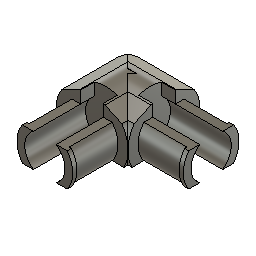
2x corner new v16 (Autodesk Fusion 360 design; units mm, degrees)
Autodesk Fusion 360 part; units mm, degrees
sketch "Sketch7" plane through (0, 0, 0) normal (0, 1, 0) x (1, 0, 0)
  circle A0 centre (0, 0) radius 16.8
  line L0 (0, 0) -> (0, -80) construction
  line L1 (0, 0) -> (100, 0) construction
  line L2 (-16.8, 16.8) -> (16.8, 16.8)
  line L3 (16.8, 16.8) -> (16.8, -16.8)
  line L4 (16.8, -16.8) -> (-16.8, -16.8)
  line L5 (-16.8, -16.8) -> (-16.8, 16.8)
  dimension "d64" = 33.6
  measures "d64" diameter of A0
ref_plane "WorkPlane2" through (0, 0, 16.8) normal (0, 0, 1) x (1, 0, 0)
ref_plane "WorkPlane3" through (16.8, 0, 0) normal (1, 0, 0) x (0, 1, 0)
sketch "Sketch1" plane through (0, 0, 16.8) normal (0, 0, 1) x (1, 0, 0)
  line L0 (-14.7788, 7.9891) -> (14.7788, 7.9891)
  circle A0 centre (0, 0) radius 12.15
  line L1 (0, 0) -> (0, 16.8) construction
  line L2 (-13.9241, 9.4) -> (13.9241, 9.4) construction
  line L3 (-14.9113, -7.7391) -> (14.9113, -7.7391)
  line L4 (-13.9241, 9.4) -> (-6.0799, 13.0535)
  line L5 (-2, 0) -> (-2, 16.6805)
  line L6 (-13.9241, -9.4) -> (-6.0799, -13.0535)
  line L7 (2, 0) -> (2, 16.6805)
  line L8 (13.9241, -9.4) -> (6.0799, -13.0535)
  line L9 (-14.9113, 7.7391) -> (14.9113, 7.7391)
  line L10 (14.7788, -7.9891) -> (-14.7788, -7.9891)
  line L11 (0, 0) -> (0, -22) construction
  line L12 (-13.9241, -9.4) -> (13.9241, -9.4) construction
  circle A1 centre (0, 0) radius 14.4
  circle A2 centre (0, 0) radius 9.4
  circle A3 centre (0, 0) radius 16.8
  circle A4 centre (0, 0) radius 12.4
  line L13 (13.9241, 9.4) -> (6.0799, 13.0535)
  line L14 (5.3353, 7.7391) -> (5.3353, 15.9303)
  line L15 (-5.3353, 7.7391) -> (-5.3353, 15.9303)
  line L16 (0, 16.8) -> (-35.6, 16.8)
  line L17 (-35.6, 16.8) -> (-35.6, -17.8)
  line L18 (-35.6, -17.8) -> (0, -17.8)
  line L19 (0, -17.8) -> (0, 16.8)
  dimension "PipeDiameter2" = 18.8
  dimension "d2" = 24.8
  dimension "d3" = 28.8
  dimension "d4" = 33.6
  dimension "d5" = 7.7391
  dimension "d6" = 7.7391
  dimension "d7" = 2
  dimension "d8" = 2
  dimension "d9" = 24.3
  dimension "d10" = 0.25
  dimension "d11" = 0.25
  dimension "d52" = 35.6
  dimension "d53" = 17.8
  measures "PipeDiameter2" diameter of A2
  measures "d2" diameter of A4
  measures "d3" diameter of A1
  measures "d4" diameter of A3
  measures "d5" distance of A0.centre L9
  measures "d6" distance of A0.centre L3
  measures "d7" distance of A0.centre L5
  measures "d8" distance of A0.centre L7
  measures "d9" diameter of A0
  measures "d10" distance of L3 L10
  measures "d11" distance of L0 L9
  measures "d52" distance of A0.centre L17
  measures "d53" distance of A0.centre L18
sketch "Sketch3" plane through (16.8, 0, 0) normal (1, 0, 0) x (0, 0, -1)
  line L0 (-14.7788, 7.9891) -> (14.7788, 7.9891)
  circle A0 centre (0, 0) radius 12.15
  line L1 (0, 0) -> (0, 16.8) construction
  line L2 (-13.9241, 9.4) -> (13.9241, 9.4) construction
  line L3 (-14.9113, -7.7391) -> (14.9113, -7.7391)
  line L4 (-13.9241, 9.4) -> (-6.0799, 13.0535)
  line L5 (-2, 0) -> (-2, 16.6805)
  line L6 (-13.9241, -9.4) -> (-6.0799, -13.0535)
  line L7 (2, 0) -> (2, 16.6805)
  line L8 (13.9241, -9.4) -> (6.0799, -13.0535)
  line L9 (-14.9113, 7.7391) -> (14.9113, 7.7391)
  line L10 (14.7788, -7.9891) -> (-14.7788, -7.9891)
  line L11 (0, 0) -> (0, -22) construction
  line L12 (-13.9241, -9.4) -> (13.9241, -9.4) construction
  circle A1 centre (0, 0) radius 14.4
  circle A2 centre (0, 0) radius 9.4
  circle A3 centre (0, 0) radius 16.8
  circle A4 centre (0, 0) radius 12.4
  line L13 (13.9241, 9.4) -> (6.0799, 13.0535)
  line L14 (5.3353, 7.7391) -> (5.3353, 15.9303)
  line L15 (-5.3353, 7.7391) -> (-5.3353, 15.9303)
  line L16 (0, 14.4) -> (35.6, 14.4)
  line L17 (35.6, 14.4) -> (35.6, -17.8)
  line L18 (35.6, -17.8) -> (0, -17.8)
  line L19 (0, -17.8) -> (0, 14.4)
  dimension "d22" = 18.8
  dimension "d23" = 24.8
  dimension "d24" = 28.8
  dimension "d25" = 33.6
  dimension "d26" = 7.7391
  dimension "d27" = 7.7391
  dimension "d28" = 2
  dimension "d29" = 2
  dimension "d30" = 24.3
  dimension "d31" = 0.25
  dimension "d32" = 0.25
  dimension "d54" = 35.6
  dimension "d55" = 17.8
  measures "d22" diameter of A2
  measures "d23" diameter of A4
  measures "d24" diameter of A1
  measures "d25" diameter of A3
  measures "d26" distance of A0.centre L9
  measures "d27" distance of A0.centre L3
  measures "d28" distance of A0.centre L5
  measures "d29" distance of A0.centre L7
  measures "d30" diameter of A0
  measures "d31" distance of L3 L10
  measures "d32" distance of L0 L9
  measures "d54" distance of A0.centre L17
  measures "d55" distance of A0.centre L18
extrude "Extrude1" add sketch "Sketch1" along normal blind 20 contours A0 L3 L9 A2 | A0 L3 L9 A2 makes body 1 at (9.0524, -2.5327, 30.1333) makes body 2 at (-5.7125, -7.4651, 30.1333)
extrude "Extrude2" add sketch "Sketch1" against normal blind 33.6 contours L0 L4 A1 A3 | L0 L9 A1 A3 | L0 A1 A4 L15 | L0 L9 A1 A4 | L3 L9 A1 A3 | L0 A0 A4 L15 | L0 A0 L9 A4 | L3 L9 A1 A4 | L0 A0 L15 | L0 A0 L9 L15 | L5 A1 A4 L15 | A0 L5 A4 L15 | A0 L3 L9 A4 | L0 A0 L5 A2 L15 | L0 A2 L15 | A0 L3 L9 A2 | A0 L5 A4 L19 | L5 A1 A4 L19 | L0 L5 A2 | L0 L5 L9 A2 | L3 L9 A2 L19 | A0 L5 A2 L19 | L7 A1 A4 L19 | A0 L7 A4 L19 | L0 L5 A2 L19 | L0 L5 L9 L19 | A0 L7 A2 L19 | A0 L7 A4 L14 | L7 A1 A4 L14 | L0 L7 A2 L19 | L0 L7 L9 L19 | L3 L9 A2 L19 | L0 A0 L7 A2 L14 | L0 A1 A4 L14 | L0 A0 A4 L14 | L0 A1 A3 L13 | L0 L7 A2 | L0 L7 L9 A2 | A0 L3 L9 A2 | L0 A0 L14 | L0 A0 L9 A4 | L0 L9 A1 A4 | L3 L9 A1 A4 | A0 L3 L9 A4 | L0 L9 A1 A3 | L3 L9 A1 A3 | L0 A2 L14 | L0 A0 L9 L14 bodies 1 2
extrude "Extrude3" cut sketch "Sketch1" against normal blind 3 contours L5 A1 A4 L15 | A0 L5 A4 L15 | L0 A0 L5 A2 L15 | L0 A2 L15 | A0 L5 A4 L19 | L5 A1 A4 L19 | L0 L5 A2 | L0 L5 L9 A2 | L3 L9 A2 L19 | A0 L5 A2 L19 | L7 A1 A4 L19 | A0 L7 A4 L19 | L0 L5 A2 L19 | L0 L5 L9 L19 | L3 L10 A2 L19 | A0 L7 A2 L19 | A0 L7 A4 L14 | L7 A1 A4 L14 | L0 L7 A2 L19 | L0 L7 L9 L19 | L3 L9 A2 L19 | L3 L10 A2 L19 | L10 A2 L19 | L0 A0 L7 A2 L14 | L0 L7 A2 | L0 L7 L9 A2 | L10 A2 L19 | L0 A2 L14 bodies 1
extrude "Extrude4" add sketch "Sketch3" along normal blind 20 separate body contours A0 L3 L9 A2 | A0 L3 L9 A2 makes body 3 at (30.1333, 7.4651, -5.7125) makes body 4 at (30.1333, -7.4651, 5.7125)
extrude "Extrude5" add sketch "Sketch3" against normal blind 33.6 contours L0 L4 A1 A3 | L0 L9 A1 A3 | L0 A1 A4 L15 | L0 L9 A1 A4 | L3 L9 A1 A3 | L0 A0 A4 L15 | L0 A0 L9 A4 | L3 L9 A1 A4 | L0 A0 L15 | L0 A0 L9 L15 | L5 A1 A4 L15 | A0 L5 A4 L15 | A0 L3 L9 A4 | L0 A0 L5 A2 L15 | L0 A2 L15 | A0 L3 L9 A2 | A0 L5 A4 L19 | L5 A1 A4 L19 | L0 L5 A2 | L0 L5 L9 A2 | L3 L9 A2 L19 | A0 L5 A2 L19 | L7 A1 A4 L19 | A0 L7 A4 L19 | L0 L5 A2 L19 | L0 L5 L9 L19 | A0 L7 A2 L19 | A0 L7 A4 L14 | L7 A1 A4 L14 | L0 L7 A2 L19 | L0 L7 L9 L19 | L3 L9 A2 L19 | L0 A0 L7 A2 L14 | L0 A1 A4 L14 | L0 A0 A4 L14 | L0 A1 A3 L13 | L0 L7 A2 | L0 L7 L9 A2 | A0 L3 L9 A2 | L0 A0 L14 | L0 A0 L9 A4 | L0 L9 A1 A4 | L3 L9 A1 A4 | A0 L3 L9 A4 | L0 L9 A1 A3 | L3 L9 A1 A3 | L0 A2 L14 | L0 A0 L9 L14 bodies 1 3 4
extrude "Extrude6" cut sketch "Sketch3" along normal blind -6.4 and the other way blind -35 contours L5 A1 A4 L15 | A0 L5 A4 L15 | L0 A0 L5 A2 L15 | L0 A2 L15 | A0 L5 A4 L19 | L5 A1 A4 L19 | L0 L5 A2 | L0 L5 L9 A2 | L3 L9 A2 L19 | A0 L5 A2 L19 | L7 A1 A4 L19 | A0 L7 A4 L19 | L0 L5 A2 L19 | L0 L5 L9 L19 | A0 L7 A2 L19 | A0 L7 A4 L14 | L7 A1 A4 L14 | L0 L7 A2 L19 | L0 L7 L9 L19 | L3 L9 A2 L19 | L0 A0 L7 A2 L14 | L0 L7 A2 | L0 L7 L9 A2 | L0 A2 L14 bodies 1
extrude "Extrude7" cut sketch "Sketch1" along normal blind -6.4 and the other way blind -32 contours L5 A1 A4 L15 | A0 L5 A4 L15 | L0 A0 L5 A2 L15 | L0 A2 L15 | A0 L5 A4 L19 | L5 A1 A4 L19 | L0 L5 A2 | L0 L5 L9 A2 | L3 L9 A2 L19 | A0 L5 A2 L19 | L7 A1 A4 L19 | A0 L7 A4 L19 | L0 L5 A2 L19 | L0 L5 L9 L19 | A0 L7 A2 L19 | A0 L7 A4 L14 | L7 A1 A4 L14 | L0 L7 A2 L19 | L0 L7 L9 L19 | L3 L9 A2 L19 | L0 A0 L7 A2 L14 | L0 L7 A2 | L0 L7 L9 A2 | L0 A2 L14 bodies 1
extrude "Extrude9" cut sketch "Sketch3" against normal blind 73 contours L7 A1 L14 L16 | A3 L16 L17 L18 L19 | A1 A3 L13 L14 L16 bodies 1
extrude "Extrude10" cut sketch "Sketch1" against normal blind 50 contours A3 L16 L17 L18 L19 | L4 A1 A3 L15 | L5 A1 A3 L15 | L5 A1 A3 L19 | L6 A1 A3 L19 | L8 A1 A3 L19 bodies 1
extrude "Extrude13" cut sketch "Sketch7" along normal mid plane 35.6 contours A0 L2 L5 bodies 1
sketch "Sketch5" plane through (36.8, 0, 0) normal (1, 0, 0) x (0, 0, -1)
  line L0 (-9.3663, -7.7391) -> (-5.3353, -7.7391)
  arc A0 (-5.3353, 7.7391) -> (-5.3353, -7.7391) centre (0, 0) ccw
  circle A1 centre (0, 0) radius 13
  line L1 (-14.9113, -7.7391) -> (14.9113, -7.7391)
  line L2 (-14.9113, 7.7391) -> (14.9113, 7.7391)
  circle A2 centre (0, 0) radius 9.4
  arc A3 (-5.3353, 7.7391) -> (-5.3353, -7.7391) centre (0, 0) ccw
  arc A4 (5.3353, -7.7391) -> (5.3353, 7.7391) centre (0, 0) ccw
  line L3 (5.3353, 7.7391) -> (5.3353, 15.9303)
  line L4 (5.3353, 7.7391) -> (5.3353, 25)
  line L5 (-16.8, 7.7391) -> (-36.8, 7.7391)
  arc A5 (-9.3663, 7.7391) -> (-9.3663, -7.7391) centre (0, 0) ccw
  line L6 (-5.3353, 7.7391) -> (-9.3663, 7.7391)
  dimension "d57" = 26
  measures "d57" diameter of A1
extrude "Extrude11" add sketch "Sketch5" along normal blind 2 contours L0 A0 L1 L2 A2 A3 A5 L6 | A1 L1 L2 A5 | A1 L1 L2 A2 A4 bodies 1
sketch "Sketch6" plane through (0, 0, 36.8) normal (0, 0, 1) x (1, 0, 0)
  arc A0 (-9.3663, 7.7391) -> (-9.3663, -7.7391) centre (0, 0) ccw
  line L0 (-9.3663, -7.7391) -> (-5.3353, -7.7391)
  arc A1 (-5.3353, 7.7391) -> (-5.3353, -7.7391) centre (0, 0) ccw
  line L1 (-5.3353, 7.7391) -> (-9.3663, 7.7391)
  circle A2 centre (0, 0) radius 13
  line L2 (-14.9113, -7.7391) -> (14.9113, -7.7391)
  line L3 (-14.9113, 7.7391) -> (14.9113, 7.7391)
  circle A3 centre (0, 0) radius 9.4
  dimension "d60" = 26
  measures "d60" diameter of A2
extrude "Extrude12" add sketch "Sketch6" along normal blind 2 contours A0 L0 A1 L1 L2 L3 A3 | A0 A2 L2 L3 | A2 L2 L3 A3 bodies 1
copy_body "Body->Comp1" [suppressed] in component "2xcorner"
equation "PipeDiameter2 = PipeDiameter + 1 mm"
equation "d2 = PipeDiameter2 + 6 mm"
equation "d3 = PipeDiameter2 + 10 mm"
equation "d4 = PipeDiameter + 15.8 mm"
equation "d5 = PipeDiameter / 2.3"
equation "d6 = PipeDiameter / 2.3"
equation "d7 = HalfOfScrewMount"
equation "d8 = HalfOfScrewMount"
equation "d9 = d2 - Tolerance * 2"
equation "d10 = Tolerance"
equation "d11 = Tolerance"
equation "PipeDiameter = 17.8 mm"
equation "Tolerance = 0.25 mm"
equation "HalfOfScrewMount = 2 mm"
equation "d22 = PipeDiameter + 1 mm"
equation "d23 = PipeDiameter2 + 6 mm"
equation "d24 = PipeDiameter2 + 10 mm"
equation "d25 = PipeDiameter + 15.8 mm"
equation "d26 = PipeDiameter / 2.3"
equation "d27 = PipeDiameter / 2.3"
equation "d28 = HalfOfScrewMount"
equation "d29 = HalfOfScrewMount"
equation "d30 = d2 - Tolerance * 2"
equation "d31 = Tolerance"
equation "d32 = Tolerance"
equation "d52 = PipeDiameter * 2"
equation "d53 = PipeDiameter"
equation "d54 = PipeDiameter * 2"
equation "d55 = PipeDiameter"
equation "d57 = PipeDiameter + 8.2 mm"
equation "d60 = PipeDiameter + 8.2 mm"
equation "d64 = PipeDiameter + 15.8 mm"
equation "d65 = ( PipeDiameter + 15.8 mm ) / 2"
equation "d66 = ( PipeDiameter + 15.8 mm ) / 2"
equation "d67 = PipeDiameter"
named bodies: "2xcorner"
